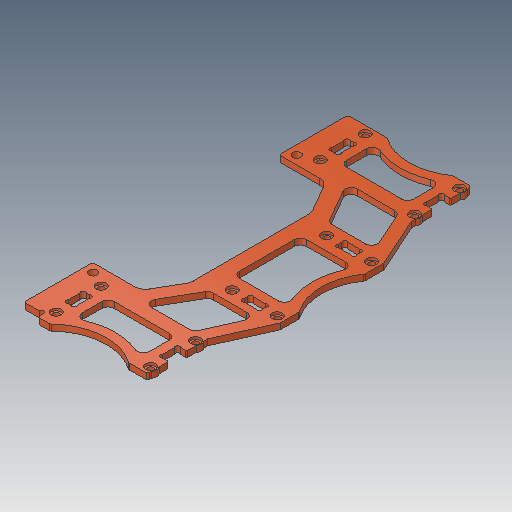
# Autodesk Inventor part: body_top
Saved by Autodesk Inventor 2019.4 (Build 234330000, 330)
## iProperties
Created: 2018-08-08
Part Number: body_top
Material: 一般
Document SubType Name: Modeling
Designer: student
Density: 1 g/cm^3
Appearance: 滑らか - 淡いオレンジ
Mass: 3.89324 g
Surface Area: 56.8915 cm^2
Volume: 3.89324 cm^3
Author: student
Autodesk Inventor part; units mm, degrees
ref_plane "YZ Plane" through (0, 0, 0) normal (1, 0, 0) x (0, 1, 0)
ref_plane "XZ Plane" through (0, 0, 0) normal (0, 1, 0) x (-1, 0, 0)
ref_plane "XY Plane" through (0, 0, 0) normal (0, 0, 1) x (1, 0, 0)
sketch "スケッチ1" plane through (0, 0, 0) normal (0, 1, 0) x (1, 0, 0)
  circle A0 centre (0, 0) radius 80 construction
  line L0 (0, 0) -> (40, 69.282) construction
  line L1 (0, 0) -> (80, 0) construction
  line L2 (0, 0) -> (40, -69.282) construction
  arc A1 (56.2792, 52.132) -> (55.2208, 52.132) centre (55.75, 51.532) ccw construction
  arc A2 (56.2792, 37.132) -> (55.2208, 37.132) centre (55.75, 36.532) ccw construction
  arc A3 (24.7792, 52.132) -> (23.7208, 52.132) centre (24.25, 51.532) ccw construction
  arc A4 (24.7792, 37.132) -> (23.7208, 37.132) centre (24.25, 36.532) ccw construction
  circle A5 centre (24.25, 51.532) radius 1.05
  circle A6 centre (24.25, 36.532) radius 1.05
  circle A7 centre (55.75, 51.532) radius 1.05
  circle A8 centre (55.75, 36.532) radius 1.05
  line L3 (57.25, 54.032) -> (51.25, 54.032)
  line L4 (54.25, 54.032) -> (57.25, 54.032) construction
  line L5 (57.25, 52.132) -> (57.25, 53.782) construction
  line L6 (54.25, 47.032) -> (57.25, 47.032) construction
  line L7 (57.25, 41.032) -> (54.25, 41.032) construction
  line L8 (57.25, 34.032) -> (54.25, 34.032) construction
  line L9 (57.25, 54.032) -> (57.25, 52.8549)
  line L10 (57.25, 47.082) -> (55.2607, 47.082)
  line L11 (54.2, 47.082) -> (54.2, 46.0214) construction
  line L12 (54.2, 40.982) -> (55.2607, 40.982) construction
  line L13 (57.25, 40.982) -> (57.25, 37.8549)
  arc A9 (55.2607, 47.082) -> (54.2, 46.0214) centre (54.7303, 46.5517) ccw
  arc A10 (54.2, 42.0427) -> (55.2607, 40.982) centre (54.7303, 41.5124) ccw
  line L14 (55.2607, 47.082) -> (54.2, 47.082) construction
  line L15 (54.2, 46.0214) -> (54.2, 42.0427)
  line L16 (54.2, 42.0427) -> (54.2, 40.982) construction
  line L17 (55.2607, 40.982) -> (57.25, 40.982)
  line L18 (64.75, 14.25) -> (64.75, 17.25) construction
  line L19 (57.25, 34.032) -> (64.75, 17.25)
  line L20 (64.75, 17.25) -> (64.75, 11.25)
  arc A11 (29.3633, 53.8238) -> (50.6808, 53.8542) centre (40, 69.282) ccw
  arc A12 (64.5722, 10.6808) -> (61.2358, 0) centre (80, 0) ccw
  line L21 (16.5, 54) -> (28.7964, 54)
  arc A13 (51.25, 54.032) -> (50.6808, 53.8542) centre (51.25, 53.032) ccw
  arc A14 (29.3633, 53.8238) -> (28.7964, 54) centre (28.7964, 53) ccw
  line L22 (22.7, 40.982) -> (23.7607, 40.982) construction
  line L23 (25.8, 40.982) -> (25.8, 42.0427) construction
  line L24 (25.8, 47.082) -> (24.7393, 47.082) construction
  line L25 (22.7, 47.082) -> (22.7, 46.0214) construction
  line L26 (25.75, 46.782) -> (25.75, 41.282) construction
  line L27 (25.75, 47.032) -> (22.75, 47.032) construction
  line L28 (25.75, 41.032) -> (22.75, 41.032) construction
  line L29 (22.75, 41.282) -> (22.75, 46.782) construction
  arc A15 (22.7, 42.0427) -> (23.7607, 40.982) centre (23.2303, 41.5124) ccw
  arc A16 (23.7607, 47.082) -> (22.7, 46.0214) centre (23.2303, 46.5517) ccw
  arc A17 (25.8, 46.0214) -> (24.7393, 47.082) centre (25.2697, 46.5517) ccw
  arc A18 (24.7393, 40.982) -> (25.8, 42.0427) centre (25.2697, 41.5124) ccw
  line L30 (22.7, 46.0214) -> (22.7, 42.0427)
  line L31 (23.7607, 47.082) -> (22.7, 47.082) construction
  line L32 (24.7393, 47.082) -> (23.7607, 47.082)
  line L33 (25.8, 46.0214) -> (25.8, 47.082) construction
  line L34 (24.7393, 40.982) -> (25.8, 40.982) construction
  line L35 (25.8, 42.0427) -> (25.8, 46.0214)
  line L36 (23.7607, 40.982) -> (24.7393, 40.982)
  line L37 (22.7, 42.0427) -> (22.7, 40.982) construction
  line L38 (0, 54.0091) -> (0, 0) construction
  arc A19 (64.5722, 10.6808) -> (64.75, 11.25) centre (63.75, 11.25) ccw
  line L39 (57.8, 17.3) -> (56.7393, 17.3) construction
  line L40 (51.7, 17.3) -> (51.7, 16.2393) construction
  line L41 (51.7, 14.2) -> (52.7607, 14.2) construction
  line L42 (57.8, 14.2) -> (57.8, 15.2607) construction
  line L43 (57.5, 14.25) -> (52, 14.25) construction
  line L44 (52, 17.25) -> (57.5, 17.25) construction
  line L45 (51.75, 17.25) -> (51.75, 14.25) construction
  line L46 (57.75, 14.25) -> (57.75, 17.25) construction
  arc A20 (52.7607, 17.3) -> (51.7, 16.2393) centre (52.2303, 16.7697) ccw
  arc A21 (51.7, 15.2607) -> (52.7607, 14.2) centre (52.2303, 14.7303) ccw
  arc A22 (56.7393, 14.2) -> (57.8, 15.2607) centre (57.2697, 14.7303) ccw
  arc A23 (57.8, 16.2393) -> (56.7393, 17.3) centre (57.2697, 16.7697) ccw
  line L47 (57.8, 16.2393) -> (57.8, 17.3) construction
  line L48 (56.7393, 17.3) -> (52.7607, 17.3)
  line L49 (57.8, 15.2607) -> (57.8, 16.2393)
  line L50 (56.7393, 14.2) -> (57.8, 14.2) construction
  line L51 (52.7607, 14.2) -> (56.7393, 14.2)
  line L52 (51.7, 15.2607) -> (51.7, 14.2) construction
  line L53 (51.7, 16.2393) -> (51.7, 15.2607)
  line L54 (52.7607, 17.3) -> (51.7, 17.3) construction
  arc A24 (62.85, 15.2208) -> (62.85, 16.2792) centre (62.25, 15.75) ccw construction
  circle A25 centre (62.25, 15.75) radius 1.05
  arc A26 (47.85, 15.2208) -> (47.85, 16.2792) centre (47.25, 15.75) ccw construction
  circle A27 centre (47.25, 15.75) radius 1.05
  line L55 (16, 53.5) -> (16, 31.6)
  line L56 (16, 53.5) -> (16.5, 54)
  line L57 (34.9199, 34.282) -> (51.4602, 34.282) construction
  arc A28 (53.2861, 33.0981) -> (51.4602, 34.282) centre (51.4602, 32.282) ccw projected
  line L58 (53.2861, 33.0981) -> (57.9706, 22.616) projected
  arc A29 (56.1447, 19.8) -> (57.9706, 22.616) centre (56.1447, 21.8) ccw projected
  line L59 (56.1447, 19.8) -> (46.5207, 19.8) construction
  arc A30 (59.9329, 8.4257) -> (59.9329, -8.4257) centre (80, 0) ccw projected
  arc A31 (59.9329, 8.4257) -> (58.0888, 11.2) centre (58.0888, 9.2) ccw projected
  line L60 (58.0888, 11.2) -> (49.25, 11.2) construction
  arc A32 (55.2208, -52.132) -> (56.2792, -52.132) centre (55.75, -51.532) ccw construction
  arc A33 (55.2208, -37.132) -> (56.2792, -37.132) centre (55.75, -36.532) ccw construction
  arc A34 (23.7208, -52.132) -> (24.7792, -52.132) centre (24.25, -51.532) ccw construction
  arc A35 (23.7208, -37.132) -> (24.7792, -37.132) centre (24.25, -36.532) ccw construction
  circle A36 centre (24.25, -51.532) radius 1.05
  circle A37 centre (24.25, -36.532) radius 1.05
  circle A38 centre (55.75, -51.532) radius 1.05
  circle A39 centre (55.75, -36.532) radius 1.05
  line L61 (57.25, -54.032) -> (51.25, -54.032)
  line L62 (54.25, -54.032) -> (57.25, -54.032) construction
  line L63 (57.25, -52.132) -> (57.25, -53.782) construction
  line L64 (54.25, -47.032) -> (57.25, -47.032) construction
  line L65 (57.25, -41.032) -> (54.25, -41.032) construction
  line L66 (57.25, -47.082) -> (55.2607, -47.082)
  line L67 (54.2, -47.082) -> (54.2, -46.0214) construction
  line L68 (54.2, -40.982) -> (55.2607, -40.982) construction
  arc A40 (54.2, -46.0214) -> (55.2607, -47.082) centre (54.7303, -46.5517) ccw
  arc A41 (55.2607, -40.982) -> (54.2, -42.0427) centre (54.7303, -41.5124) ccw
  line L69 (55.2607, -47.082) -> (54.2, -47.082) construction
  line L70 (54.2, -46.0214) -> (54.2, -42.0427)
  line L71 (54.2, -42.0427) -> (54.2, -40.982) construction
  line L72 (55.2607, -40.982) -> (57.25, -40.982)
  line L73 (64.75, -14.25) -> (64.75, -17.25) construction
  line L74 (57.25, -34.032) -> (64.75, -17.25)
  line L75 (64.75, -17.25) -> (64.75, -11.25)
  arc A42 (50.6808, -53.8542) -> (27.0293, -55.7226) centre (40, -69.282) ccw
  arc A43 (61.2358, 0) -> (64.5722, -10.6808) centre (80, 0) ccw
  arc A44 (50.6808, -53.8542) -> (51.25, -54.032) centre (51.25, -53.032) ccw
  line L76 (22.7, -40.982) -> (23.7607, -40.982) construction
  line L77 (25.8, -40.982) -> (25.8, -42.0427) construction
  line L78 (25.8, -47.082) -> (24.7393, -47.082) construction
  line L79 (22.7, -47.082) -> (22.7, -46.0214) construction
  line L80 (25.75, -46.782) -> (25.75, -41.282) construction
  line L81 (25.75, -47.032) -> (22.75, -47.032) construction
  line L82 (25.75, -41.032) -> (22.75, -41.032) construction
  line L83 (22.75, -41.282) -> (22.75, -46.782) construction
  arc A45 (23.7607, -40.982) -> (22.7, -42.0427) centre (23.2303, -41.5124) ccw
  arc A46 (22.7, -46.0214) -> (23.7607, -47.082) centre (23.2303, -46.5517) ccw
  arc A47 (24.7393, -47.082) -> (25.8, -46.0214) centre (25.2697, -46.5517) ccw
  arc A48 (25.8, -42.0427) -> (24.7393, -40.982) centre (25.2697, -41.5124) ccw
  line L84 (22.7, -46.0214) -> (22.7, -42.0427)
  line L85 (23.7607, -47.082) -> (22.7, -47.082) construction
  line L86 (24.7393, -47.082) -> (23.7607, -47.082)
  line L87 (25.8, -46.0214) -> (25.8, -47.082) construction
  line L88 (24.7393, -40.982) -> (25.8, -40.982) construction
  line L89 (25.8, -42.0427) -> (25.8, -46.0214)
  line L90 (23.7607, -40.982) -> (24.7393, -40.982)
  line L91 (22.7, -42.0427) -> (22.7, -40.982) construction
  arc A49 (64.75, -11.25) -> (64.5722, -10.6808) centre (63.75, -11.25) ccw
  line L92 (51.7, -17.3) -> (51.7, -16.2393) construction
  line L93 (51.7, -14.2) -> (52.7607, -14.2) construction
  line L94 (57.8, -14.2) -> (57.8, -15.2607) construction
  arc A50 (51.7, -16.2393) -> (52.7607, -17.3) centre (52.2303, -16.7697) ccw
  arc A51 (52.7607, -14.2) -> (51.7, -15.2607) centre (52.2303, -14.7303) ccw
  arc A52 (57.8, -15.2607) -> (56.7393, -14.2) centre (57.2697, -14.7303) ccw
  arc A53 (56.7393, -17.3) -> (57.8, -16.2393) centre (57.2697, -16.7697) ccw
  line L95 (57.8, -16.2393) -> (57.8, -17.3) construction
  line L96 (57.8, -15.2607) -> (57.8, -16.2393)
  line L97 (56.7393, -14.2) -> (57.8, -14.2) construction
  line L98 (52.7607, -14.2) -> (56.7393, -14.2)
  line L99 (51.7, -15.2607) -> (51.7, -14.2) construction
  line L100 (51.7, -16.2393) -> (51.7, -15.2607)
  arc A54 (62.85, -16.2792) -> (62.85, -15.2208) centre (62.25, -15.75) ccw construction
  circle A55 centre (62.25, -15.75) radius 1.05
  arc A56 (47.85, -16.2792) -> (47.85, -15.2208) centre (47.25, -15.75) ccw construction
  circle A57 centre (47.25, -15.75) radius 1.05
  arc A58 (58.0888, -11.2) -> (59.9329, -8.4257) centre (58.0888, -9.2) ccw projected
  line L101 (49.25, -11.2) -> (58.0888, -11.2) construction
  arc A59 (31.5743, 49.2149) -> (28.8, 47.3709) centre (30.8, 47.3709) ccw projected
  arc A60 (31.5743, 49.2149) -> (48.4257, 49.2149) centre (40, 69.282) ccw projected
  arc A61 (51.2, 47.3709) -> (48.4257, 49.2149) centre (49.2, 47.3709) ccw projected
  line L102 (51.2, 47.3709) -> (51.2, 40.782) projected
  arc A62 (49.2, 38.782) -> (51.2, 40.782) centre (49.2, 40.782) ccw projected
  line L103 (49.2, 38.782) -> (30.8, 38.782) projected
  arc A63 (28.8, 40.782) -> (30.8, 38.782) centre (30.8, 40.782) ccw projected
  line L104 (28.8, 40.782) -> (28.8, 47.3709) projected
  arc A64 (28.8, -47.3709) -> (31.5743, -49.2149) centre (30.8, -47.3709) ccw
  arc A65 (48.4257, -49.2149) -> (31.5743, -49.2149) centre (40, -69.282) ccw
  arc A66 (48.4257, -49.2149) -> (51.2, -47.3709) centre (49.2, -47.3709) ccw
  line L105 (51.2, -47.3709) -> (51.2, -40.782)
  arc A67 (51.2, -40.782) -> (49.2, -38.782) centre (49.2, -40.782) ccw
  line L106 (49.2, -38.782) -> (30.8, -38.782)
  arc A68 (30.8, -38.782) -> (28.8, -40.782) centre (30.8, -40.782) ccw
  line L107 (28.8, -40.782) -> (28.8, -47.3709)
  line L108 (58.0888, 11.2) -> (45, 11.2)
  line L109 (58.0888, -11.2) -> (45, -11.2)
  line L110 (43, -9.2) -> (43, 9.2)
  arc A69 (45, 11.2) -> (43, 9.2) centre (45, 9.2) ccw
  arc A70 (43, -9.2) -> (45, -11.2) centre (45, -9.2) ccw
  line L111 (56.1447, 19.8) -> (44.9304, 19.8)
  line L112 (43.1984, 20.8) -> (37.1466, 31.282)
  line L113 (38.8786, 34.282) -> (51.4602, 34.282)
  arc A71 (38.8786, 34.282) -> (37.1466, 31.282) centre (38.8786, 32.282) ccw
  arc A72 (43.1984, 20.8) -> (44.9304, 19.8) centre (44.9304, 21.8) ccw
  line L114 (57.25, -34.032) -> (54.25, -34.032) construction
  line L115 (34.9199, -34.282) -> (51.4602, -34.282) construction
  arc A73 (51.4602, -34.282) -> (53.2861, -33.0981) centre (51.4602, -32.282) ccw
  line L116 (53.2861, -33.0981) -> (57.9706, -22.616)
  arc A74 (57.9706, -22.616) -> (56.1447, -19.8) centre (56.1447, -21.8) ccw
  line L117 (56.1447, -19.8) -> (46.5207, -19.8) construction
  line L118 (56.1447, -19.8) -> (44.9304, -19.8)
  line L119 (43.1984, -20.8) -> (37.1466, -31.282)
  line L120 (38.8786, -34.282) -> (51.4602, -34.282)
  arc A75 (37.1466, -31.282) -> (38.8786, -34.282) centre (38.8786, -32.282) ccw
  arc A76 (44.9304, -19.8) -> (43.1984, -20.8) centre (44.9304, -21.8) ccw
  line L121 (16.5, -54) -> (21.05, -54)
  line L122 (22.55, -54) -> (22.55, -55.5)
  line L123 (22.55, -55.5) -> (23.05, -56)
  arc A77 (22.55, -54) -> (21.05, -54) centre (21.8, -54) ccw
  arc A78 (57.25, 50.2092) -> (57.25, 52.8549) centre (55.75, 51.532) ccw
  arc A79 (57.25, 35.2092) -> (57.25, 37.8549) centre (55.75, 36.532) ccw
  line L124 (57.25, 52.8549) -> (57.25, 50.2092) construction
  line L125 (57.25, 50.2092) -> (57.25, 47.082)
  line L126 (57.25, 37.8549) -> (57.25, 35.2092) construction
  line L127 (57.25, 35.2092) -> (57.25, 34.032)
  arc A80 (57.25, -52.8549) -> (57.25, -50.2092) centre (55.75, -51.532) ccw
  arc A81 (57.25, -37.8549) -> (57.25, -35.2092) centre (55.75, -36.532) ccw
  line L128 (57.25, -40.982) -> (57.25, -37.8549)
  line L129 (57.25, -35.2092) -> (57.25, -34.032)
  line L130 (57.25, -54.032) -> (57.25, -52.8549)
  line L131 (57.25, -50.2092) -> (57.25, -47.082)
  line L132 (52.7607, -17.3) -> (56.7393, -17.3)
  line L133 (23.05, -56) -> (26.3381, -56)
  line L134 (16.5, -54) -> (16, -53.5)
  arc A82 (26.3381, -56) -> (27.0293, -55.7226) centre (26.3381, -55) ccw
  line L135 (16, -53.5) -> (16, -31.6)
  line L136 (16, -31) -> (30, -31) construction
  arc A83 (30, -31) -> (33.0311, -29.25) centre (30, -27.5) ccw construction
  line L137 (33.0311, -29.25) -> (37.5311, -21.4558) construction
  arc A84 (37.5311, -21.4558) -> (38, -19.7058) centre (34.5, -19.7058) ccw construction
  line L138 (38, -19.7058) -> (38, 18.866) construction
  arc A85 (38, 18.866) -> (37.5311, 20.616) centre (34.5, 18.866) ccw construction
  line L139 (32.5463, 29.25) -> (37.5311, 20.616) construction
  arc A86 (32.5463, 29.25) -> (29.5152, 31) centre (29.5152, 27.5) ccw construction
  line L140 (16, 31) -> (29.5152, 31) construction
  line L141 (16.5, -31.1) -> (30, -31.1)
  arc A87 (30, -31.1) -> (33.1177, -29.3) centre (30, -27.5) ccw
  line L142 (33.1177, -29.3) -> (37.6177, -21.5058)
  arc A88 (37.6177, -21.5058) -> (38.1, -19.7058) centre (34.5, -19.7058) ccw
  line L143 (38.1, -19.7058) -> (38.1, 18.866)
  arc A89 (38.1, 18.866) -> (37.6177, 20.666) centre (34.5, 18.866) ccw
  line L144 (37.6177, 20.666) -> (32.6329, 29.3)
  arc A90 (32.6329, 29.3) -> (29.5152, 31.1) centre (29.5152, 27.5) ccw
  line L145 (29.5152, 31.1) -> (16.5, 31.1)
  line L146 (16, -31.6) -> (16.5, -31.1)
  line L147 (16.5, 31.1) -> (16, 31.6)
  circle A91 centre (19, 34) radius 1.4
  circle A92 centre (19, -34) radius 1.4
  circle A93 centre (19, -34) radius 2 construction
  circle A94 centre (19, 34) radius 2 construction
  point P0 (50.9332, 54.032)
  point P1 (64.75, 10.9332)
  point P2 (16, 23.0729)
  point P3 (16, 54)
  point P4 (32.05, 0)
  point P5 (50.9332, -54.032)
  point P6 (64.75, -10.9332)
  point P7 (26.7454, -56)
  point P8 (16, -54)
  point P9 (16, -31.1)
  point P10 (16, 31.1)
  dimension "d2" = 160
  dimension "d3" = 60
  dimension "d4" = 60
  dimension "d7" = 2.1
  dimension "d8" = 0.05
  dimension "d9" = 0.05
  dimension "d10" = 3.05
  dimension "d11" = 0.75
  dimension "d13" = 1
  dimension "d14" = 1
  dimension "d15" = 6
  dimension "d16" = 0.05
  dimension "d17" = 0.05
  dimension "d18" = 0.05
  dimension "d19" = 0.05
  dimension "d20" = 0.75
  dimension "d21" = 1
  dimension "d22" = 6
  dimension "d23" = 0.05
  dimension "d24" = 0.05
  dimension "d25" = 0.05
  dimension "d26" = 0.05
  dimension "d27" = 0.75
  dimension "d28" = 2.1
  dimension "d29" = 16
  dimension "d31" = 6.95
  dimension "d35" = 54
  dimension "d36" = 0.5
  dimension "d37" = 0.5
  dimension "d42" = 2
  dimension "d45" = 2
  dimension "d46" = 0.75
  dimension "d49" = 0.5
  dimension "d53" = 2
  dimension "d63" = 0.5
  dimension "d64" = 2
  dimension "d65" = 0.5
  dimension "d66" = 0.5
  dimension "d67" = 1
  dimension "d68" = 56
  dimension "d71" = 0.1
  dimension "d72" = 0.5
  dimension "d73" = 0.5
  dimension "d74" = 0.5
  dimension "d75" = 0.5
  dimension "d76" = 4.9
  dimension "d77" = 4.9
  dimension "d78" = 2.8
  constraints: 238 end point, 135 point on circle, 131 symmetric about line, 73 centre point, 37 parallel, 28 perpendicular, 22 point on line, 18 horizontal, 17 tangent, 15 coincident, 15 equal radius, 14 collinear, 8 vertical, 4 concentric, 51 other
  measures "d2" diameter of A0
  measures "d3" angle of L1 L0
  measures "d4" angle of L1 L2
  measures "d7" diameter of A8
  measures "d8" distance between parallel lines of L10 L6
  measures "d9" distance between parallel lines of L12 L7
  measures "d10" distance between parallel lines of L11 L9
  measures "d11" radius of A9
  measures "d13" radius of A13
  measures "d14" radius of A14
  measures "d15" distance of L3.start L3.end
  measures "d16" distance between parallel lines of L22 L28
  measures "d18" distance between parallel lines of L24 L27
  measures "d19" distance between parallel lines of L25 L29
  measures "d20" radius of A15
  measures "d21" radius of A19
  measures "d22" distance of L18.end L20.end
  measures "d23" distance between parallel lines of L41 L43
  measures "d24" distance between parallel lines of L40 L45
  measures "d25" distance between parallel lines of L39 L44
  measures "d26" distance between parallel lines of L42 L46
  measures "d27" radius of A20
  measures "d28" diameter of A25
  measures "d29" distance between parallel lines of L38 L55
  measures "d31" distance of L13.start L19.start
  measures "d35" distance between parallel lines of L21 L1
  measures "d36" distance of L55.start point (16, 54)
  measures "d37" distance of L21.start point (16, 54)
  measures "d42" radius of A69
  measures "d45" radius of A71
  measures "d46" radius of A77
  measures "d49" distance from line of L123.end L122
  measures "d53" radius of A78
  measures "d63" distance from line of L122.end L133
  measures "d64" distance between parallel lines of L121 L133
  measures "d65" distance of L121.start point (16, -54)
  measures "d66" distance of L134.end point (16, -54)
  measures "d67" radius of A82
  measures "d68" distance between parallel lines of L1 L133
  measures "d71" distance between parallel lines of L136 L141
  measures "d72" distance of L135.end point (16, -31.1)
  measures "d73" distance of L141.start point (16, -31.1)
  measures "d74" distance of L145.end point (16, 31.1)
  measures "d75" distance of L55.end point (16, 31.1)
  measures "d76" distance between parallel lines of L144 L112
  measures "d77" distance between parallel lines of L110 L143
  measures "d78" diameter of A92
extrude "押し出し1" add sketch "スケッチ1" along normal blind 2
sketch "スケッチ2" plane through (0, 2, 0) normal (0, 1, 0) x (1, 0, 0)
  line L0 (0, 0) -> (29.2462, 0)
  circle A0 centre (55.75, 51.532) radius 1.05 projected
  circle A1 centre (55.75, 51.532) radius 1.7
  circle A2 centre (24.25, 51.532) radius 1.05 projected
  circle A3 centre (24.25, 51.532) radius 1.7
  circle A4 centre (24.25, 36.532) radius 1.05 projected
  circle A5 centre (24.25, 36.532) radius 1.7
  circle A6 centre (55.75, 36.532) radius 1.05 projected
  circle A7 centre (55.75, 36.532) radius 1.7
  circle A8 centre (47.25, 15.75) radius 1.05 projected
  circle A9 centre (47.25, 15.75) radius 1.7
  circle A10 centre (62.25, 15.75) radius 1.05 projected
  circle A11 centre (62.25, 15.75) radius 1.7
  circle A12 centre (55.75, -51.532) radius 1.05
  circle A13 centre (55.75, -51.532) radius 1.7
  circle A14 centre (24.25, -51.532) radius 1.05
  circle A15 centre (24.25, -51.532) radius 1.7
  circle A16 centre (24.25, -36.532) radius 1.05
  circle A17 centre (24.25, -36.532) radius 1.7
  circle A18 centre (55.75, -36.532) radius 1.05
  circle A19 centre (55.75, -36.532) radius 1.7
  circle A20 centre (47.25, -15.75) radius 1.05
  circle A21 centre (47.25, -15.75) radius 1.7
  circle A22 centre (62.25, -15.75) radius 1.05
  circle A23 centre (62.25, -15.75) radius 1.7
  dimension "d54" = 3.4
  constraints: 18 centre point, 12 coincident, 12 symmetric about line, 5 equal radius, 2 end point, 1 horizontal, 12 other
  measures "d54" diameter of A3
extrude "押し出し2" cut sketch "スケッチ2" against normal blind 0.8 contours A0 | A1 | A2 | A3 | A4 | A5 | A6 | A7 | A8 | A9 | A10 | A11 | A12 | A13 | A14 | A15 | A16 | A17 | A18 | A19 | A20 | A21 | A22 | A23
chamfer "面取り1" distance 0.5 angle 45 2 edges at (57.25, 1, 54.032) (57.25, 1, -54.032)
chamfer "面取り2" distance 0.25 angle 45 4 edges at (57.25, 1, -47.082) (57.25, 1, -40.982) (57.25, 1, 40.982) (57.25, 1, 47.082)
